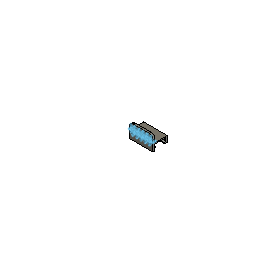
KeyboardAdapter (Autodesk Fusion 360 archive; units mm, degrees)
design "interactLatch_laatch"
Autodesk Fusion 360 part; units mm, degrees
note: some values were not read from the file. Chosen so that the rebuilt part matches the saved one: which face or edge a step refers to; which pieces of a blend or face edit are solid.
sketch "Sketch1" plane through (0, 21, 0) normal (0, 1, 0) x (-1, 0, 0)
  line L0 (12, 5) -> (-12, 5)
  line L1 (-12, 5) -> (-12, -4)
  line L2 (-12, -4) -> (12, -4)
  line L3 (12, -4) -> (12, 5)
  line L4 (0, 5) -> (0, -4) construction
  line L5 (-13.1, -4) -> (13.1, -4)
  line L6 (13.1, -4) -> (13.1, 5)
  line L7 (13.1, 5) -> (-13.1, 5)
  line L8 (-13.1, 5) -> (-13.1, -4)
  line L9 (-13.1, -4) -> (13.1, 5) construction
  line L10 (13.1, -4) -> (-13.1, 5) construction
  point P0 (0, 0.5)
  dimension "d189" = 26.2
  constraint midpoint L0 L4.start
  constraint midpoint L2 L4.end
  constraint horizontal L5
  constraint perpendicular L5 L6
  constraint parallel L5 L7
  constraint parallel L6 L8
  constraint coincident L9 P0
  constraint coincident L10 P0
  constraint midpoint L4 P0
  measures "d189" distance of L6.end L7.end
extrude "Extrude1" add sketch "Sketch1" along normal blind 2
extrude "Extrude2" add 3 faces at (4, 21.6667, -4) (-12.3667, 21.6667, -4) (12.7333, 21.6667, -4) along direction (0, 0, -1) blind 2
sketch "Sketch2" plane through (0, 21, 0) normal (0, -1, 0) x (1, 0, 0)
  line L0 (13.1, -6) -> (13.1, 5)
  line L1 (13.1, 5) -> (-13.1, 5)
  line L2 (-13.1, 5) -> (-13.1, -6)
  line L3 (-13.1, -6) -> (13.1, -6)
  line L4 (-13.1, -6) -> (13.1, -6)
  line L5 (13.1, -6) -> (13.1, -4)
  line L6 (13.1, -4) -> (-13.1, -4)
  line L7 (-13.1, -4) -> (-13.1, -6)
  dimension "d194" = 2
  constraint horizontal L4
  constraint vertical L5
  constraint horizontal L6
  constraint vertical L7
  constraint coincident L2.end L3.start
  measures "d194" distance of L2.end L6.end
extrude "Extrude3" add sketch "Sketch2" along normal blind 6 contours L0 L2 L3 L4 L5 L6 L7
sketch "Sketch3" plane through (0, 0, -4) normal (0, 0, 1) x (1, 0, 0)
  line L0 (13.1, 21) -> (-13.1, 21)
  line L1 (-13.1, 21) -> (-13.1, 15)
  line L2 (-13.1, 15) -> (13.1, 15)
  line L3 (13.1, 15) -> (13.1, 21)
  line L4 (-9.9, 18.9) -> (9.9, 18.9)
  line L5 (9.9, 18.9) -> (9.9, 15.1)
  line L6 (9.9, 15.1) -> (-9.9, 15.1)
  line L7 (-9.9, 15.1) -> (-9.9, 18.9)
  line L8 (-9.9, 18.9) -> (9.9, 15.1) construction
  line L9 (9.9, 18.9) -> (-9.9, 15.1) construction
  point P0 (0, 17)
  dimension "d197" = 19.8
  dimension "d198" = 3.8
  constraint horizontal L4
  constraint perpendicular L4 L5
  constraint parallel L4 L6
  constraint parallel L5 L7
  constraint coincident L8 P0
  constraint coincident L9 P0
  measures "d197" distance of L5.end L6.end
  measures "d198" distance of L4.end L5.end
extrude "Extrude4" add sketch "Sketch3" along normal blind 1 contours L4 L5 L6 L7
extrude "Extrude5" add 1 faces at (-4.3667, 21.6667, 5) along direction (0, 0, 1) blind 1
sketch "Sketch4" plane through (0, 21, 0) normal (0, -1, 0) x (1, 0, 0)
  line L0 (-13.1, -4) -> (13.1, -4)
  line L1 (13.1, -4) -> (13.1, 6)
  line L2 (13.1, 6) -> (-13.1, 6)
  line L3 (-13.1, 6) -> (-13.1, -4)
  line L4 (-13.1, 6) -> (13.1, 6)
  line L5 (13.1, 6) -> (13.1, 5)
  line L6 (13.1, 5) -> (-13.1, 5)
  line L7 (-13.1, 5) -> (-13.1, 6)
  line L8 (-9.9, 5) -> (9.9, 5)
  line L9 (9.9, 5) -> (9.9, 6)
  line L10 (9.9, 6) -> (-9.9, 6)
  line L11 (-9.9, 6) -> (-9.9, 5)
  line L12 (-9.9, 5) -> (9.9, 6) construction
  line L13 (9.9, 5) -> (-9.9, 6) construction
  point P0 (0, 5.5)
  dimension "d203" = 1
  dimension "d204" = 19.8
  constraint horizontal L4
  constraint vertical L5
  constraint horizontal L6
  constraint vertical L7
  constraint coincident L2.end L3.start
  constraint horizontal L8
  constraint perpendicular L8 L9
  constraint parallel L8 L10
  constraint parallel L9 L11
  constraint coincident L12 P0
  constraint coincident L13 P0
  measures "d203" distance of L2.end L6.end
  measures "d204" distance of L9.end L10.end
extrude "Extrude6" add sketch "Sketch4" along normal blind 5 contours L2 L4 L6 L8 L9 L10 L11
sketch "Sketch5" plane through (9.9, 0, 0) normal (1, 0, 0) x (0, 0, -1)
  line L0 (-5, 21) -> (-6, 21)
  line L1 (-6, 21) -> (-6, 16)
  line L2 (-6, 16) -> (-5, 16)
  line L3 (-5, 16) -> (-5, 21)
  line L4 (-5, 16) -> (-5, 18.8)
  line L5 (-5, 18.8) -> (-4, 18.8)
  line L6 (-4, 18.8) -> (-5, 16)
  dimension "d207" = 2.8
  constraint coincident L2.end L3.start
  constraint perpendicular L2 L4
  constraint perpendicular L4 L5
  measures "d207" distance of L2.end L4.end
extrude "Extrude7" add sketch "Sketch5" against normal blind 19.8 contours L3 L4 L5 L6
extrude "Extrude8" cut 1 faces at (-13.1, 22.3333, -1.3333) along direction (1, 0, 0) blind 3.2
extrude "Extrude9" cut 1 faces at (13.1, 22.3333, -1.3333) along direction (-1, 0, 0) blind 3.2
sketch "sketch 2179" plane through (0, 23, 0) normal (0, 1, 0) x (-1, 0, 0)
  line L0 (9.9, 4) -> (9.9, 6)
  line L1 (9.9, 4) -> (9.9, 6)
  line L2 (9.9, 6) -> (-9.9, 6)
  line L3 (9.9, 6) -> (-9.9, 6)
  line L4 (-9.9, 6) -> (-9.9, 4)
  line L5 (-9.9, 6) -> (-9.9, 4)
  line L6 (-9.9, 4) -> (9.9, 4)
extrude "Extrude10" add sketch "sketch 2179" along normal blind 5
fillet "Fillet1" radius 3 2 edges at (9.9, 28, 5) (-9.9, 28, 5)
sketch "sketch 2204" plane through (0, 0, 6) normal (0, 0, 1) x (1, 0, 0)
  line L0 (3.6, 20) -> (5, 22)
  line L1 (2, 22) -> (3.6, 20)
  line L2 (2, 21.5) -> (2, 22)
  line L3 (3.6, 19.5) -> (2, 21.5)
  line L4 (5, 21.5) -> (3.6, 19.5)
  line L5 (5, 22) -> (5, 21.5)
  line L6 (-3.4, 20) -> (-2, 22)
  line L7 (-5, 22) -> (-3.4, 20)
  line L8 (-5, 21.5) -> (-5, 22)
  line L9 (-3.4, 19.5) -> (-5, 21.5)
  line L10 (-2, 21.5) -> (-3.4, 19.5)
  line L11 (-2, 22) -> (-2, 21.5)
  line L12 (-6.9, 22.5) -> (-5.5, 24.5)
  line L13 (-8.5, 24.5) -> (-6.9, 22.5)
  line L14 (-8.5, 24) -> (-8.5, 24.5)
  line L15 (-6.9, 22) -> (-8.5, 24)
  line L16 (-5.5, 24) -> (-6.9, 22)
  line L17 (-5.5, 24.5) -> (-5.5, 24)
  line L18 (0.1, 22.5) -> (1.5, 24.5)
  line L19 (-1.5, 24.5) -> (0.1, 22.5)
  line L20 (-1.5, 24) -> (-1.5, 24.5)
  line L21 (0.1, 22) -> (-1.5, 24)
  line L22 (1.5, 24) -> (0.1, 22)
  line L23 (1.5, 24.5) -> (1.5, 24)
  line L24 (7.1, 22.5) -> (8.5, 24.5)
  line L25 (5.5, 24.5) -> (7.1, 22.5)
  line L26 (5.5, 24) -> (5.5, 24.5)
  line L27 (7.1, 22) -> (5.5, 24)
  line L28 (8.5, 24) -> (7.1, 22)
  line L29 (8.5, 24.5) -> (8.5, 24)
  line L30 (3.6, 25) -> (5, 27)
  line L31 (2, 27) -> (3.6, 25)
  line L32 (2, 26.5) -> (2, 27)
  line L33 (3.6, 24.5) -> (2, 26.5)
  line L34 (5, 26.5) -> (3.6, 24.5)
  line L35 (5, 27) -> (5, 26.5)
  line L36 (-3.4, 25) -> (-2, 27)
  line L37 (-5, 27) -> (-3.4, 25)
  line L38 (-5, 26.5) -> (-5, 27)
  line L39 (-3.4, 24.5) -> (-5, 26.5)
  line L40 (-2, 26.5) -> (-3.4, 24.5)
  line L41 (-2, 27) -> (-2, 26.5)
  line L42 (-6.9, 24.5) -> (-8.5, 26.5)
  line L43 (-5.5, 26.5) -> (-6.9, 24.5)
  line L44 (-5.5, 27) -> (-5.5, 26.5)
  line L45 (-6.9, 25) -> (-5.5, 27)
  line L46 (-8.5, 27) -> (-6.9, 25)
  line L47 (-8.5, 26.5) -> (-8.5, 27)
  line L48 (0.1, 25) -> (1.5, 27)
  line L49 (-1.5, 27) -> (0.1, 25)
  line L50 (-1.5, 26.5) -> (-1.5, 27)
  line L51 (0.1, 24.5) -> (-1.5, 26.5)
  line L52 (1.5, 26.5) -> (0.1, 24.5)
  line L53 (1.5, 27) -> (1.5, 26.5)
  line L54 (7.1, 25) -> (8.5, 27)
  line L55 (5.5, 27) -> (7.1, 25)
  line L56 (5.5, 26.5) -> (5.5, 27)
  line L57 (7.1, 24.5) -> (5.5, 26.5)
  line L58 (8.5, 26.5) -> (7.1, 24.5)
  line L59 (8.5, 27) -> (8.5, 26.5)
  line L60 (3.6, 22.5) -> (5, 24.5)
  line L61 (2, 24.5) -> (3.6, 22.5)
  line L62 (2, 24) -> (2, 24.5)
  line L63 (3.6, 22) -> (2, 24)
  line L64 (5, 24) -> (3.6, 22)
  line L65 (5, 24.5) -> (5, 24)
  line L66 (-3.4, 22.5) -> (-2, 24.5)
  line L67 (-5, 24.5) -> (-3.4, 22.5)
  line L68 (-5, 24) -> (-5, 24.5)
  line L69 (-3.4, 22) -> (-5, 24)
  line L70 (-2, 24) -> (-3.4, 22)
  line L71 (-2, 24.5) -> (-2, 24)
  line L72 (-6.9, 20) -> (-5.5, 22)
  line L73 (-8.5, 22) -> (-6.9, 20)
  line L74 (-8.5, 21.5) -> (-8.5, 22)
  line L75 (-6.9, 19.5) -> (-8.5, 21.5)
  line L76 (-5.5, 21.5) -> (-6.9, 19.5)
  line L77 (-5.5, 22) -> (-5.5, 21.5)
  line L78 (0.1, 20) -> (1.5, 22)
  line L79 (-1.5, 22) -> (0.1, 20)
  line L80 (-1.5, 21.5) -> (-1.5, 22)
  line L81 (0.1, 19.5) -> (-1.5, 21.5)
  line L82 (1.5, 21.5) -> (0.1, 19.5)
  line L83 (1.5, 22) -> (1.5, 21.5)
  line L84 (7.1, 20) -> (8.5, 22)
  line L85 (5.5, 22) -> (7.1, 20)
  line L86 (5.5, 21.5) -> (5.5, 22)
  line L87 (7.1, 19.5) -> (5.5, 21.5)
  line L88 (8.5, 21.5) -> (7.1, 19.5)
  line L89 (8.5, 22) -> (8.5, 21.5)
extrude "Extrude11" add sketch "sketch 2204" along normal blind 0.2
sketch "Sketch6" plane through (9.9, 0, 0) normal (1, 0, 0) x (0, 0, -1)
  line L0 (-4, 25) -> (-6, 25)
  line L1 (-6, 25) -> (-6, 16)
  line L2 (-6, 16) -> (-5, 16)
  line L3 (-5, 16) -> (-4, 18.8)
  line L4 (-4, 18.8) -> (-5, 18.8)
  line L5 (-5, 18.8) -> (-5, 21)
  line L6 (-5, 21) -> (4, 21)
  line L7 (4, 21) -> (4, 18.9)
  line L8 (4, 18.9) -> (3, 18.9)
  line L9 (3, 18.9) -> (3, 15.1)
  line L10 (3, 15.1) -> (4, 15.1)
  line L11 (4, 15.1) -> (4, 15)
  line L12 (4, 15) -> (6, 15)
  line L13 (6, 15) -> (6, 23)
  line L14 (6, 23) -> (-4, 23)
  line L15 (-4, 23) -> (-4, 25)
  line L16 (3.5, 18.9) -> (3, 17.7406)
  constraint midpoint L8 L16.start
  constraint coincident L9 L16.end
extrude "Extrude12" cut sketch "Sketch6" against normal blind 19.8 contours L8 L9 L16
extrude "Extrude13" cut 1 faces at (3.3, 23, -2.6667) along direction (0, -1, 0) blind 1
extrude "Extrude14" cut 1 faces at (-3.3, 15, -4.6667) along direction (0, 1, 0) blind 0.1
extrude "Extrude15" cut 1 faces at (3.3, 15.1, -5.3333) along direction (0, 1, 0) blind 2
move_face "OffsetFaces2" offset -0.4 1 faces at (-2.3, 24, 4)
move_face "OffsetFaces3" offset -0.8 3 faces at (-3.3, 19.6, -4) (3.3, 17.5271, -3) (-3.3, 18.5135, -3.3333)
